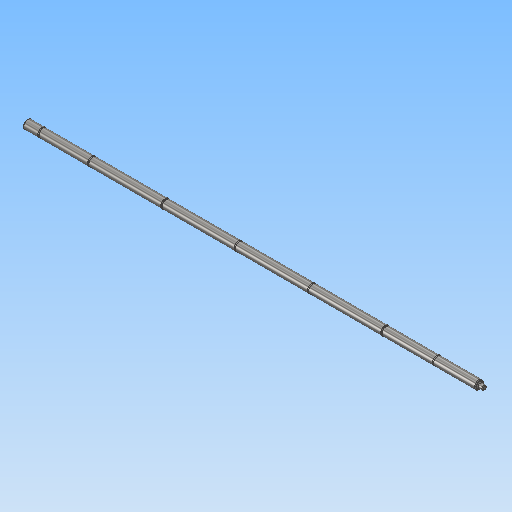
# Autodesk Inventor part: Selection_Selector Shaft
Saved by Autodesk Inventor 2018.1 (Build 221171000, 171)
## iProperties
Created: 2019-02-07
Part Number: Selection_Selector Shaft
Material: Steel, Mild
Document SubType Name: Modeling
Designer: James
Density: 7.85 g/cm^3
Appearance: Semi-Polished
Mass: 68.5068 g
Surface Area: 59.2125 cm^2
Volume: 8.72698 cm^3
Author: James
Autodesk Inventor part; units mm, degrees
ref_plane "YZ Plane" through (0, 0, 0) normal (1, 0, 0) x (0, 1, 0)
ref_plane "XZ Plane" through (0, 0, 0) normal (0, 1, 0) x (-1, 0, 0)
ref_plane "XY Plane" through (0, 0, 0) normal (0, 0, 1) x (1, 0, 0)
derived "Selection_Skeleton.ipt"
ref_plane "Ground" through (0, 0, 0) normal (0, 1, 0) x (-1, 0, 0)
ref_plane "LHS inner" through (0, 0, 0) normal (1, 0, 0) x (0, 1, 0)
ref_plane "RHS inner" through (300, 0, 0) normal (1, 0, 0) x (0, 1, 0)
ref_plane "Lane 1" through (50, 0, 0) normal (1, 0, 0) x (0, 1, 0)
ref_plane "Lane 2" through (100, 0, 0) normal (1, 0, 0) x (0, 1, 0)
ref_plane "Lane 3" through (150, 0, 0) normal (1, 0, 0) x (0, 1, 0)
ref_plane "Lane 4" through (200, 0, 0) normal (1, 0, 0) x (0, 1, 0)
ref_plane "Lane 5" through (250, 0, 0) normal (1, 0, 0) x (0, 1, 0)
ref_plane "Back" through (0, 0, 0) normal (0, 0, 1) x (1, 0, 0)
sketch "Sketch1" plane through (0, 0, 0) normal (1, 0, 0) x (0, 1, 0)
  circle A0 centre (0, 0) radius 3
  dimension "d1" = 6
  constraints: 1 centre point, 1 coincident
  measures "d1" diameter of A0
extrude "Extrusion1" add sketch "Sketch1" along normal up to surface (300 mm away)
sketch "Sketch5" plane through (0, 0, 0) normal (0, 0, 1) x (1, 0, 0)
  line L0 (49, 3) -> (49.8, 3)
  line L1 (49.8, 3) -> (49.8, 2.85)
  line L2 (49.8, 2.85) -> (49, 2.85)
  line L3 (49, 2.85) -> (49, 3)
  line L4 (-60, 0) -> (360, 0) projected
  line L5 (50, 8.5367) -> (50, -4.9228) projected
  line L6 (0, 3) -> (0, -3) projected
  point P0 (0, 0)
  dimension "d22" = 2.85
  dimension "d23" = 0.8
  dimension "d24" = 1
  constraints: 8 end point, 2 parallel, 1 horizontal, 1 horizontal alignment, 1 perpendicular
  measures "d22" distance between parallel lines of L2 L4
  measures "d23" distance of L0.start L0.end
  measures "d24" distance between parallel lines of L5 L3
revolve "Revolution2" cut sketch "Sketch5" angle 360 about axis through (-10, 0, 0) along (1, 0, 0)
pattern_linear "Rectangular Pattern2" count 5 spacing 50 along (1, 0, 0) of "Revolution2"
sketch "Sketch6" plane through (300, 0, 0) normal (1, 0, 0) x (0, 0, -1)
  circle A0 centre (0, 0) radius 3 projected
extrude "extrusion 2" add sketch "Sketch6" along normal blind 17
sketch "Sketch7" plane through (0, 0, 0) normal (-1, 0, 0) x (0, 0, 1)
  circle A0 centre (0, 0) radius 3 projected
extrude "remove 5 opp" cut sketch "Sketch7" against normal blind 5
chamfer "Chamfer3" distance 0.5 angle 45 1 edges at (5, -3, 0)
sketch "Sketch8" plane through (0, 0, 0) normal (0, 0, 1) x (1, 0, 0)
  line L0 (15, 3) -> (15.8, 3)
  line L1 (15.8, 3) -> (15.8, 2.85)
  line L2 (15.8, 2.85) -> (15, 2.85)
  line L3 (15, 2.85) -> (15, 3)
  line L4 (-59, 0) -> (354, 0) projected
  line L5 (5, -2.5) -> (5, 2.5) projected
  line L6 (5.5, 3) -> (5.5, -3) projected
  point P0 (0, 0)
  dimension "d39" = 2.85
  dimension "d40" = 0.8
  dimension "d41" = 10
  constraints: 8 end point, 2 parallel, 1 horizontal, 1 horizontal alignment, 1 perpendicular
  measures "d39" distance between parallel lines of L2 L4
  measures "d40" distance of L0.start L0.end
  measures "d41" distance between parallel lines of L3 L5
revolve "Revolution3" cut sketch "Sketch8" angle 360 about axis through (-10, 0, 0) along (1, 0, 0)
ref_plane "mid plane" through (150, 0, 0) normal (1, 0, 0) x (0, 1, 0)
mirror "Mirror1" about plane through (150, 0, 0) normal (1, 0, 0) of "Revolution3"
sketch "Sketch10" plane through (0, 0, 0) normal (0, 1, 0) x (-1, 0, 0)
  line L0 (-317, 3) -> (-313.5, 3)
  line L1 (-313.5, 3) -> (-313.5, 1.5)
  line L2 (-313.5, 1.5) -> (-317, 1.5)
  line L3 (-317, 1.5) -> (-317, 3)
  line L4 (64.027, 0) -> (-384.1619, 0) projected
  line L5 (-285, 3) -> (-285, -3) projected
  line L6 (-317, 3) -> (-317, -3) projected
  point P0 (0, 0)
  dimension "d43" = 1.5
  dimension "d44" = 3.5
  constraints: 8 end point, 2 coincident, 2 parallel, 1 horizontal, 1 perpendicular
  measures "d43" distance between parallel lines of L4 L2
  measures "d44" distance of L0.start L0.end
revolve "Revolution4" cut sketch "Sketch10" angle 360 about axis through (-10, 0, 0) along (1, 0, 0)
chamfer "Chamfer4" distance 0.5 angle 45 2 edges at (317, 0, -1.5) (313.5, 0, 3)
fillet "Fillet1" radius 0.5 1 edges at (313.5, 0, -1.5)
body "Solid1"
